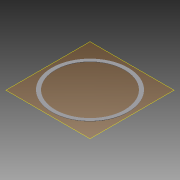
# Autodesk Inventor part: top
Saved by Autodesk Inventor 2015 SP1 (Build 190203100, 203)
## iProperties
Created: 2015-02-17
Part Number: top
Material: Wood (Birch)
Document SubType Name: Modeling
Designer: Jostein
Density: 0.55 g/cm^3
Appearance: Birch - Natural Polished
Author: Jostein
Autodesk Inventor part; units mm, degrees
ref_plane "YZ Plane" through (0, 0, 0) normal (1, 0, 0) x (0, 1, 0)
ref_plane "XZ Plane" through (0, 0, 0) normal (0, 1, 0) x (-1, 0, 0)
ref_plane "XY Plane" through (0, 0, 0) normal (0, 0, 1) x (1, 0, 0)
ref_plane "Work Plane1" through (0, 0, 0) normal (0, 0, 1) x (1, 0, 0)
sketch "Sketch1" plane through (0, 0, 0) normal (0, 0, 1) x (1, 0, 0)
  circle A0 centre (-290, 0) radius 274 projected
  circle A1 centre (-290, 0) radius 244
  point P0 (0, 0)
  dimension "d0" = 30
  constraints: 1 centre point
  measures "d0" radial gap between concentric circles of A0 A1
extrude "Extrusion1" add sketch "Sketch1" along normal blind 3
body "Solid1"
